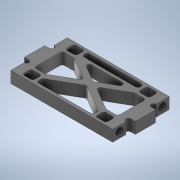
# Autodesk Inventor part: Head_diagonal
Saved by Autodesk Inventor 2020 (Build 240168000, 168)
## iProperties
Part Number: Head_diagonal
Material: アセタール樹脂、黒
Document SubType Name: Modeling
Designer: Masato Kubotera
Density: 1.425 g/cm^3
Appearance: 滑らか - 黒
Description: POM T5
Mass: 3.69423 g
Surface Area: 34.5802 cm^2
Volume: 2.59244 cm^3
Author: Masato Kubotera
Autodesk Inventor part; units mm, degrees
ref_plane "YZ Plane" through (0, 0, 0) normal (1, 0, 0) x (0, 1, 0)
ref_plane "XZ Plane" through (0, 0, 0) normal (0, 1, 0) x (-1, 0, 0)
ref_plane "XY Plane" through (0, 0, 0) normal (0, 0, 1) x (1, 0, 0)
sketch "スケッチ1" plane through (0, 0, 0) normal (0, 0, 1) x (1, 0, 0)
  line L0 (-12.5, -22.5) -> (-12.5, 22.5)
  line L1 (-12.5, 22.5) -> (12.5, 22.5)
  line L2 (12.5, 22.5) -> (12.5, -22.5)
  line L3 (12.5, -22.5) -> (-12.5, -22.5)
  line L4 (-12.5, -22.5) -> (12.5, 22.5) construction
  line L5 (-12.5, 22.5) -> (12.5, -22.5) construction
  line L6 (0, -22.5) -> (0, 22.5) construction
  line L7 (-12.5, 0) -> (12.5, 0) construction
  line L8 (-4.5, -22.5) -> (-4.5, -24.5)
  line L9 (-4.5, -24.5) -> (4.5, -24.5)
  arc A0 (-4.5, -22.5) -> (-6.6, -22.5) centre (-5.55, -22.5) ccw
  line L10 (-9.5, -22.5) -> (-9.5, -18.5) construction
  line L11 (-11.5, -22.5) -> (-11.5, -18.5) construction
  line L12 (-11.5, -18.5) -> (-7.5, -18.5) construction
  line L13 (-7.5, -18.5) -> (-7.5, -22.5) construction
  line L14 (4.5, -22.5) -> (4.5, -24.5)
  arc A1 (6.6, -22.5) -> (4.5, -22.5) centre (5.55, -22.5) ccw
  line L15 (9.5, -22.5) -> (9.5, -18.5) construction
  line L16 (11.5, -22.5) -> (11.5, -18.5) construction
  line L17 (11.5, -18.5) -> (7.5, -18.5) construction
  line L18 (7.5, -18.5) -> (7.5, -22.5) construction
  line L19 (-11.25, -11.25) -> (-8.75, -11.25) construction
  line L20 (-8.75, -11.25) -> (-8.75, 11.25)
  line L21 (-8.75, 11.25) -> (-11.25, 11.25) construction
  line L22 (-11.25, 11.25) -> (-11.25, -11.25)
  line L23 (-11.25, -11.25) -> (-8.75, 11.25) construction
  line L24 (-8.75, -11.25) -> (-11.25, 11.25) construction
  arc A2 (-11.25, -11.25) -> (-8.75, -11.25) centre (-10, -11.25) ccw
  arc A3 (-8.75, 11.25) -> (-11.25, 11.25) centre (-10, 11.25) ccw
  line L25 (-10, -12.5) -> (-10, 12.5) construction
  line L26 (-8.5, -13.75) -> (-10.5, -13.75)
  line L27 (-11.5, -14.75) -> (-11.5, -17.5)
  line L28 (-10.5, -18.5) -> (-8.5, -18.5)
  line L29 (-7.5, -17.5) -> (-7.5, -14.75)
  line L30 (-7.5, -13.75) -> (-11.5, -18.5) construction
  line L31 (-11.5, -13.75) -> (-7.5, -18.5) construction
  arc A4 (-11.5, -17.5) -> (-10.5, -18.5) centre (-10.5, -17.5) ccw
  arc A5 (-8.5, -18.5) -> (-7.5, -17.5) centre (-8.5, -17.5) ccw
  arc A6 (-7.5, -14.75) -> (-8.5, -13.75) centre (-8.5, -14.75) ccw
  arc A7 (-10.5, -13.75) -> (-11.5, -14.75) centre (-10.5, -14.75) ccw
  line L32 (-6.25, -17.5) -> (-6.25, -13.6166)
  line L33 (-6.1164, -13.1173) -> (-0.8664, -4.007)
  line L34 (-5.25, -18.5) -> (0, -18.5)
  line L35 (-7.5, -6.7731) -> (-7.5, 0)
  line L36 (-5.6336, -7.2724) -> (-1.7304, -0.4993)
  arc A8 (-7.5, -6.7731) -> (-5.6336, -7.2724) centre (-6.5, -6.7731) ccw
  arc A9 (-6.1164, -13.1173) -> (-6.25, -13.6166) centre (-5.25, -13.6166) ccw
  arc A10 (-6.25, -17.5) -> (-5.25, -18.5) centre (-5.25, -17.5) ccw
  line L37 (-8.5, -14.75) -> (0, 0) construction
  line L38 (-7.5, 6.7731) -> (-7.5, 0)
  line L39 (-5.6336, 7.2724) -> (-1.7304, 0.4993)
  arc A11 (-5.6336, 7.2724) -> (-7.5, 6.7731) centre (-6.5, 6.7731) ccw
  arc A12 (-1.7304, -0.4993) -> (-1.7304, 0.4993) centre (-2.5969, 0) ccw
  line L40 (-12.5, 0) -> (12.5, 0)
  line L41 (6.25, -17.5) -> (6.25, -13.6166)
  line L42 (6.1164, -13.1173) -> (0.8664, -4.007)
  line L43 (5.25, -18.5) -> (0, -18.5)
  arc A13 (6.25, -13.6166) -> (6.1164, -13.1173) centre (5.25, -13.6166) ccw
  arc A14 (5.25, -18.5) -> (6.25, -17.5) centre (5.25, -17.5) ccw
  arc A15 (0.8664, -4.007) -> (-0.8664, -4.007) centre (0, -4.5063) ccw
  line L44 (8.5, -13.75) -> (10.5, -13.75)
  line L45 (11.5, -14.75) -> (11.5, -17.5)
  line L46 (10.5, -18.5) -> (8.5, -18.5)
  line L47 (7.5, -17.5) -> (7.5, -14.75)
  arc A16 (10.5, -18.5) -> (11.5, -17.5) centre (10.5, -17.5) ccw
  arc A17 (8.5, -13.75) -> (7.5, -14.75) centre (8.5, -14.75) ccw
  arc A18 (11.5, -14.75) -> (10.5, -13.75) centre (10.5, -14.75) ccw
  arc A19 (7.5, -17.5) -> (8.5, -18.5) centre (8.5, -17.5) ccw
  line L48 (1.7304, -0.4993) -> (8.3576, -11.9993)
  line L49 (9.224, -12.5) -> (10.25, -12.5)
  line L50 (11.25, -11.5) -> (11.25, 0)
  line L51 (1.7304, 0.4993) -> (8.3576, 11.9993)
  line L52 (9.224, 12.5) -> (10.25, 12.5)
  line L53 (11.25, 11.5) -> (11.25, 0)
  arc A20 (1.7304, 0.4993) -> (1.7304, -0.4993) centre (2.5969, 0) ccw
  arc A21 (8.3576, -11.9993) -> (9.224, -12.5) centre (9.224, -11.5) ccw
  arc A22 (10.25, -12.5) -> (11.25, -11.5) centre (10.25, -11.5) ccw
  arc A23 (11.25, 11.5) -> (10.25, 12.5) centre (10.25, 11.5) ccw
  arc A24 (9.224, 12.5) -> (8.3576, 11.9993) centre (9.224, 11.5) ccw
  point P0 (-10, 0)
  point P1 (4.5, -22.5)
  point P2 (6.6, -22.5)
  point P3 (4.5, -22.5)
  point P4 (-9.5, -16.125)
  point P5 (-9.5, -16.125)
  point P6 (0, -2.5035)
  point P7 (1.4427, 0)
  point P8 (8.6461, -12.5)
  point P9 (11.25, -12.5)
  point P10 (8.6461, 12.5)
  point P11 (11.25, 12.5)
  point P12 (-11.25, 0)
  point P13 (1.5969, 0)
  point P14 (-1.5969, 0)
  point P15 (-8.75, 0)
  dimension "d0" = 4
  dimension "d1" = 4
  dimension "d2" = 1.05
  dimension "d3" = 19
  dimension "d4" = 9
  dimension "d5" = 25
  dimension "d7" = 2
  dimension "d8" = 45
  dimension "d9" = 1.25
  dimension "d10" = 25
  dimension "d11" = 1.25
  dimension "d35" = 1
  dimension "d36" = 4
  dimension "d37" = 1.25
  dimension "d38" = 1.25
  dimension "d39" = 1.25
  dimension "d41" = 1
  dimension "d42" = 1
  dimension "d43" = 1
  dimension "d44" = 1
  dimension "d45" = 1.25
  dimension "d46" = 1.25
  dimension "d47" = 1.25
  dimension "d48" = 2.5
  dimension "d49" = 1.25
  dimension "d50" = 1
  constraints: 106 end point, 52 point on circle, 34 symmetric about line, 28 tangent, 27 point on line, 25 centre point, 12 midpoint, 9 perpendicular, 8 equal radius, 8 parallel, 4 vertical, 2 collinear, 2 horizontal, 19 other
  measures "d0" distance of L10.end L10.start
  measures "d1" distance of L11.end L12.end
  measures "d2" radius of A0
  measures "d3" distance of L15.start L10.start
  measures "d4" distance of L8.end L9.end
  measures "d5" distance of L2.end L0.start
  measures "d7" distance of L8.start L8.end
  measures "d8" distance of L0.start L0.end
  measures "d9" radius of A2
  measures "d10" distance of L25.start L25.end
  measures "d11" horizontal distance of L7.start L19.start
  measures "d35" radius of A4
  measures "d36" distance between parallel lines of L29 L27
  measures "d37" distance edge to line of A2 L26
  measures "d38" distance between parallel lines of L32 L29
  measures "d39" distance from line of L35 L19.end
  measures "d41" radius of A8
  measures "d42" radius of A9
  measures "d43" radius of A12
  measures "d44" radius of A15
  measures "d45" distance between parallel lines of L33 L37
  measures "d46" distance between parallel lines of L37 L36
  measures "d47" distance between parallel lines of L44 L49
  measures "d48" distance between parallel lines of L42 L48
  measures "d49" distance between parallel lines of L2 L50
  measures "d50" radius of A20
extrude "押し出し1" add sketch "スケッチ1" along normal blind 5 contours L0 L40 L22 A2 L20 L35 A8 L36 A12 A20 L48 A21 L49 A22 L50 L2 L3 A1 A0 | L3 L14 L9 L8
sketch "スケッチ2" plane through (-12.5, -22.5, 0) normal (0, -1, 0) x (1, 0, 0)
  line L0 (12.5, 5) -> (12.5, 0)
  line L1 (0, 0) -> (5.9, 0) projected
  line L2 (8, 5) -> (5.9, 5) projected
  point P0 (3, 2.5)
  point P1 (22, 2.5)
  point P2 (17, 5)
  dimension "d22" = 2.5
  dimension "d30" = 19
  constraints: 2 end point, 1 point on line, 1 symmetric about line, 1 vertical
  measures "d22" distance from line of L1 point (3, 2.5)
  measures "d30" distance of point (22, 2.5) point (3, 2.5)
hole "穴1" at (-9.5, -22.5, 2.5) at (9.5, -22.5, 2.5) direction (0, 1, 0) diameter 3.4587 depth 5 tip angle 118 thread size "M4x0.5" class "6H" standard "ISO Metric profile"
mirror "ミラー1" about plane through (-11.25, 0, 0) normal (0, 1, 0)
equation "\"d37\" = d11"
equation "\"d38\" = d11"
equation "\"d39\" = d11"
equation "\"d30\" = d3"
